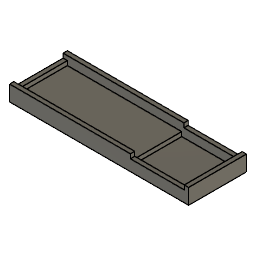
Canal - Middle plate v10 (Autodesk Fusion 360 design; units mm, degrees)
Autodesk Fusion 360 part; units mm, degrees
note: some values were not read from the file. Set by a fixed rule: which sketch regions a step uses.
sketch "Sketch1" plane through (0, 0, 0) normal (0, 0, 1) x (1, 0, 0)
  line L0 (38.5, 25) -> (80, 25)
  line L1 (80, 25) -> (80, 11.6)
  line L2 (80, 11.6) -> (38.5, 11.6)
  line L3 (38.5, 11.6) -> (38.5, 25)
  dimension "d1" = 41.5
  dimension "d2" = 13.4
  constraint horizontal L0
  constraint vertical L1
  constraint horizontal L2
  constraint vertical L3
  measures "d1" distance of L1.end L2.end
  measures "d2" distance of L0.start L2.end
extrude "Extrude1" add sketch "Sketch1" along normal blind 0.6
sketch "Sketch2" plane through (0, 0, 0.6) normal (0, 0, 1) x (-1, 0, 0)
  line L0 (-38.5, -11.6) -> (-80, -11.6)
  line L1 (-80, -11.6) -> (-80, -25)
  line L2 (-80, -25) -> (-38.5, -25)
  line L3 (-38.5, -25) -> (-38.5, -11.6)
  line L4 (-39.5, -24) -> (-79, -24)
  line L5 (-79, -12.6) -> (-39.5, -12.6)
  line L6 (-39.5, -12.6) -> (-39.5, -24)
  line L7 (-80, -18.3) -> (-38.5, -18.3) construction
  line L8 (-66.5, -24) -> (-66.5, -25)
  line L9 (-79, -24) -> (-79, -12.6)
  line L10 (-59.25, -25) -> (-59.25, -11.6) construction
  line L11 (-66.5, -12.6) -> (-66.5, -11.6)
  line L12 (-39.5, -24) -> (-38.5, -24)
  line L13 (-39.5, -12.6) -> (-38.5, -12.6)
  line L14 (-79, -12.6) -> (-79, -11.6)
  line L15 (-79, -24) -> (-79, -25)
  dimension "d5" = 1
  dimension "d6" = 1
  dimension "d12" = 27
  constraint horizontal L4
  constraint horizontal L5
  constraint vertical L6
  constraint midpoint L1 L7.start
  constraint midpoint L3 L7.end
  constraint symmetric L4 L5 L7
  constraint coincident L4 L8.start
  constraint coincident L2 L8.end
  constraint perpendicular L2 L8
  constraint perpendicular L5 L9
  constraint midpoint L2 L10.start
  constraint midpoint L0 L10.end
  constraint symmetric L6 L9 L10
  constraint symmetric L7 L8.start L11.start
  constraint symmetric L7 L8.end L11.end
  constraint coincident L3 L12.end
  constraint perpendicular L3 L12
  constraint coincident L3 L13.end
  constraint perpendicular L3 L13
  constraint coincident L0 L14.end
  constraint perpendicular L0 L14
  constraint coincident L2 L15.end
  constraint perpendicular L2 L15
  measures "d5" distance of L3 L6
  measures "d6" distance of L2 L4
  measures "d12" distance of L4.start L8.start
extrude "Extrude14" add sketch "Sketch2" along normal blind 3 contours L0 L3 L5 L11 L13 | L0 L1 L2 L9 L14 L15 | L2 L3 L4 L8 L12
extrude "Extrude9" add sketch "Sketch2" along normal blind 2 contours L0 L5 L11 L14 | L3 L6 L12 L13 | L2 L4 L8 L15
sketch "Sketch7" plane through (0, 0, 0.6) normal (0, 0, 1) x (-1, 0, 0)
  line L0 (-39.5, -12.6) -> (-79, -12.6)
  line L1 (-79, -12.6) -> (-79, -24)
  line L2 (-79, -24) -> (-39.5, -24)
  line L3 (-66, -24) -> (-39.5, -24)
  line L4 (-39.5, -24) -> (-39.5, -12.6)
  line L5 (-39.5, -12.6) -> (-66, -12.6)
  line L6 (-66, -12.6) -> (-66, -24)
  line L7 (-39.5, -24) -> (-39.5, -12.6)
  constraint horizontal L3
  constraint vertical L4
  constraint horizontal L5
  constraint vertical L6
  constraint coincident L0.start L4.end
  constraint coincident L2 L3.start
extrude "Extrude17" add sketch "Sketch7" along normal blind 1 contours L0 L2 L3 L4 L5 L6 L7
